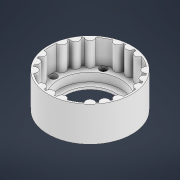
# Autodesk Inventor part: Bottom
Saved by Autodesk Inventor 2021 (Build 250183000, 183)
## iProperties
Created: 2022-10-05
Part Number: Bottom
Material: Tworzywo sztuczne ABS
Document SubType Name: Modeling
Designer: MicnedSQ
Density: 1.06 g/cm^3
Appearance: Gładki — biały
Author: MicnedSQ
Autodesk Inventor part; units mm, degrees
ref_plane "YZ Plane" through (0, 0, 0) normal (1, 0, 0) x (0, 1, 0)
ref_plane "XZ Plane" through (0, 0, 0) normal (0, 1, 0) x (-1, 0, 0)
ref_plane "XY Plane" through (0, 0, 0) normal (0, 0, 1) x (1, 0, 0)
sketch "Szkic1" plane through (0, 0, 0) normal (0, 1, 0) x (-1, 0, 0)
  circle A0 centre (0, 0) radius 35
  dimension "d0" = 70
  constraints: 1 centre point, 1 coincident
  measures "d0" diameter of A0
extrude "Wyciągnięcie proste1" add sketch "Szkic1" along normal blind 9
sketch "Szkic2" plane through (0, 9, 0) normal (0, 1, 0) x (1, 0, 0)
  circle A0 centre (-30.5, 0) radius 3
  point P0 (0, 0)
  dimension "d3" = 6
  dimension "d4" = 30.5
  constraints: 1 centre point
  measures "d3" diameter of A0
  measures "d4" distance of point (0, 0) A0.centre
extrude "Wyciągnięcie proste2" cut sketch "Szkic2" against normal blind 5
sketch "Szkic3" plane through (-30.5, 4, 0) normal (0, 1, 0) x (1, 0, 0)
  circle A0 centre (0, 0) radius 1.75
  point P0 (30.5, 0)
  dimension "d7" = 3.5
  constraints: 1 centre point
  measures "d7" diameter of A0
extrude "Wyciągnięcie proste3" cut sketch "Szkic3" against normal up to surface (4 mm away)
pattern_circular "Szyk kołowy1" count 6 over 360 about axis through (0, 0, 0) along (0, 1, 0) of "Wyciągnięcie proste2", "Wyciągnięcie proste3"
sketch "Szkic4" plane through (0, 9, 0) normal (0, 1, 0) x (1, 0, 0)
  circle A0 centre (0, 0) radius 33.5
  circle A1 centre (0, 0) radius 35 projected
  circle A2 centre (0, 0) radius 35
  dimension "d13" = 67
  dimension "d16" = 70
  constraints: 2 centre point, 2 coincident
  measures "d13" diameter of A0
  measures "d16" diameter of A2
extrude "Wyciągnięcie proste4" add sketch "Szkic4" along normal blind 20
sketch "Szkic5" plane through (0, 9, 0) normal (0, 1, 0) x (1, 0, 0)
  circle A0 centre (0, 0) radius 26
  dimension "d17" = 52
  constraints: 1 centre point, 1 coincident
  measures "d17" diameter of A0
extrude "Wyciągnięcie proste5" cut sketch "Szkic5" against normal blind 7
sketch "Szkic6" plane through (0, 2, 0) normal (0, 1, 0) x (1, 0, 0)
  circle A0 centre (0, 0) radius 21
  dimension "d20" = 42
  constraints: 1 centre point, 1 coincident
  measures "d20" diameter of A0
extrude "Wyciągnięcie proste6" cut sketch "Szkic6" against normal up to surface (2 mm away)
sketch "Szkic7" plane through (0, 9, 0) normal (0, 1, 0) x (1, 0, 0)
  arc A0 (16.75, 29.0119) -> (-16.75, 29.0119) centre (0, 0) ccw projected
  arc A1 (-3.4952, 33.3172) -> (3.4952, 33.3172) centre (0, 33.5) ccw
  dimension "d23" = 7
  constraints: 5 point on circle, 1 centre point
  measures "d23" diameter of A1
extrude "Wyciągnięcie proste7" add sketch "Szkic7" along normal up to surface (20 mm away)
pattern_circular "Szyk kołowy2" count 24 over 360 about axis through (0, 9, 0) along (0, 1, 0) of "Wyciągnięcie proste7" skipped copies 3 7 11 15 19 23
